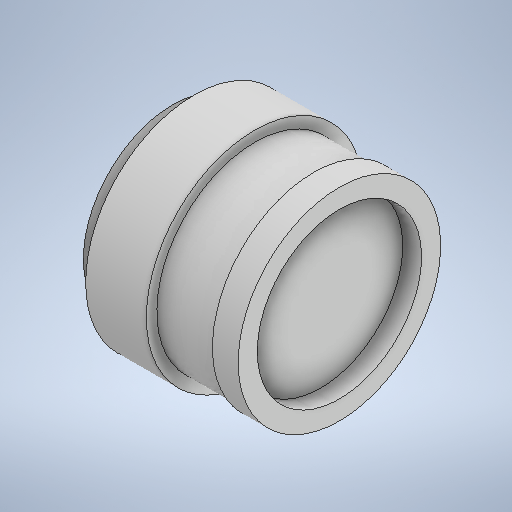
# Autodesk Inventor part: obiektyw
Saved by Autodesk Inventor 2025.1 (Build 291241000, 241)
## iProperties
Created: 2024-11-26
Part Number: obiektyw
Material: Ogólny
Document SubType Name: Modeling
Designer: PC
Density: 1 g/cm^3
Appearance: Domyślna
Author: PC
Autodesk Inventor part; units mm, degrees
ref_plane "YZ Plane" through (0, 0, 0) normal (1, 0, 0) x (0, 1, 0)
ref_plane "XZ Plane" through (0, 0, 0) normal (0, 1, 0) x (-1, 0, 0)
ref_plane "XY Plane" through (0, 0, 0) normal (0, 0, 1) x (1, 0, 0)
sketch "Szkic1" plane through (0, 0, 0) normal (0, 0, 1) x (1, 0, 0)
  line L0 (0, 0) -> (0, 25)
  line L1 (0, 25) -> (6, 25)
  line L2 (6, 25) -> (6, 30.35)
  line L3 (6, 30.35) -> (23, 30.35)
  line L4 (23, 30.35) -> (23, 27.4)
  line L5 (23, 27.4) -> (39.5, 27.4)
  line L6 (39.5, 27.4) -> (39.5, 28.35)
  line L7 (39.5, 28.35) -> (46.7, 28.35)
  line L8 (46.7, 28.35) -> (46.7, 23)
  line L9 (46.7, 0) -> (0, 0)
  line L10 (46.7, 23) -> (41.45, 23)
  line L11 (41.45, 23) -> (41.45, 0)
  dimension "d0" = 25
  dimension "d1" = 6
  dimension "d3" = 30.35
  dimension "d4" = 17
  dimension "d5" = 27.4
  dimension "d6" = 16.5
  dimension "d7" = 7.2
  dimension "d8" = 28.35
  dimension "d10" = 5.25
  dimension "d11" = 23
  constraints: 24 end point, 7 perpendicular, 2 horizontal, 2 vertical, 1 parallel, 1 point on line
  measures "d0" distance of L0.start L0.end
  measures "d1" distance of L0.end L1.end
  measures "d3" vertical distance of L0.start L2.end
  measures "d4" distance of L2.end L3.end
  measures "d5" vertical distance of L0.start L4.end
  measures "d6" distance of L4.end L5.end
  measures "d7" distance of L6.end L7.end
  measures "d8" distance between parallel lines of L9 L7
  measures "d10" distance of L8.end L10.end
  measures "d11" distance of L10.end L11.end
revolve "Obrót1" add sketch "Szkic1" angle 360 about axis through (46.7, 0, 0) along (-1, 0, 0)
